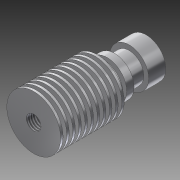
# Autodesk Inventor part: SINK-B
Saved by Autodesk Inventor 2014 SP1 (Build 180222100, 222)
## iProperties
Created: 2017-07-08
Part Number: SINK-B
Material: Типовые
Document SubType Name: Modeling
Designer: Stepan
Density: 1 g/cm^3
Appearance: Алюминий — полированный
Author: Stepan
Autodesk Inventor part; units mm, degrees
ref_plane "YZ Plane" through (0, 0, 0) normal (1, 0, 0) x (0, 1, 0)
ref_plane "XZ Plane" through (0, 0, 0) normal (0, 1, 0) x (-1, 0, 0)
ref_plane "XY Plane" through (0, 0, 0) normal (0, 0, 1) x (1, 0, 0)
sketch "Эскиз1" plane through (0, 0, 0) normal (0, 0, 1) x (1, 0, 0)
  line L0 (0, 46) -> (8, 46) construction
  line L1 (8, 46) -> (8, 39)
  line L2 (8, 39) -> (6, 39)
  line L3 (6, 39) -> (6, 33)
  line L4 (6, 33) -> (8, 33)
  line L5 (8, 33) -> (8, 30)
  line L6 (0, 0) -> (11.0018, 0)
  line L7 (11.0018, 0) -> (11.0018, 1)
  line L8 (11.0018, 1) -> (4, 1)
  line L9 (4, 1) -> (4, 2.5)
  line L10 (0, 2.5) -> (11, 2.5) construction
  line L11 (4, 2.5) -> (11, 2.5)
  line L12 (11, 2.5) -> (11, 3.5)
  line L13 (11, 3.5) -> (4, 3.5)
  line L14 (4, 3.5) -> (4, 5)
  line L15 (4, 21) -> (4, 22.5)
  line L16 (4, 22.5) -> (11, 22.5)
  line L17 (11, 22.5) -> (11, 23.5)
  line L18 (11, 23.5) -> (4, 23.5)
  line L19 (4, 23.5) -> (4, 25)
  line L20 (4, 25) -> (11, 25)
  line L21 (11, 25) -> (11, 26)
  line L22 (11, 26) -> (4, 26)
  line L23 (4, 26) -> (4, 27.5)
  line L24 (4, 27.5) -> (8, 27.5)
  line L25 (8, 27.5) -> (8, 28.5)
  line L26 (8, 28.5) -> (4, 28.5)
  line L27 (4, 28.5) -> (4, 30)
  line L28 (4, 30) -> (8, 30)
  line L29 (8, 46) -> (0, 46)
  line L30 (0, 0) -> (0, 46) construction
  line L31 (0, 0) -> (0, 46)
  line L32 (4, 21) -> (11, 21)
  line L33 (11, 21) -> (11, 20)
  line L34 (11, 20) -> (4, 20)
  line L35 (4, 20) -> (4, 18.5)
  line L36 (4, 18.5) -> (11, 18.5)
  line L37 (11, 18.5) -> (11, 17.5)
  line L38 (11, 17.5) -> (4, 17.5)
  line L39 (4, 17.5) -> (4, 16)
  line L40 (4, 16) -> (11, 16)
  line L41 (11, 16) -> (11, 15)
  line L42 (11, 15) -> (4, 15)
  line L43 (4, 15) -> (4, 13.5)
  line L44 (4, 13.5) -> (11, 13.5)
  line L45 (11, 13.5) -> (11, 12.5)
  line L46 (11, 12.5) -> (4, 12.5)
  line L47 (4, 12.5) -> (4, 11)
  line L48 (4, 11) -> (11, 11)
  line L49 (11, 11) -> (11, 10)
  line L50 (11, 10) -> (4, 10)
  line L51 (4, 10) -> (4, 8.5)
  line L52 (4, 8.5) -> (11, 8.5)
  line L53 (11, 8.5) -> (11, 7.5)
  line L54 (11, 7.5) -> (4, 7.5)
  line L55 (4, 7.5) -> (4, 6)
  line L56 (4, 6) -> (11, 6)
  line L57 (11, 6) -> (11, 5)
  line L58 (11, 5) -> (4, 5)
  dimension "d0" = 46
  dimension "d1" = 8
  dimension "d2" = 7
  dimension "d4" = 6
  dimension "d5" = 3
  dimension "d9" = 1
  dimension "d10" = 1.5
  dimension "d11" = 11
  dimension "d12" = 1
  dimension "d13" = 1.5
  dimension "d27" = 1.5
  dimension "d28" = 1
  dimension "d29" = 1.5
  dimension "d30" = 1.5
  dimension "d31" = 1
  dimension "d32" = 1
  dimension "d33" = 1.5
  dimension "d34" = 1
  dimension "d35" = 1.5
  dimension "d36" = 1
  dimension "d37" = 1.5
  dimension "d38" = 1
  dimension "d39" = 1.5
  dimension "d40" = 1
  dimension "d41" = 1.5
  dimension "d42" = 1
  dimension "d43" = 1.5
  constraints: 118 end point, 24 parallel, 20 perpendicular, 7 collinear
  measures "d0" distance of L6.start L0.start
  measures "d1" distance of L0.start L0.end
  measures "d2" distance of L0.end L1.end
  measures "d4" distance of L2.end L3.end
  measures "d5" distance of L4.end L5.end
  measures "d9" distance of L6.end L7.end
  measures "d10" distance of L8.end L9.end
  measures "d11" distance of L10.start L10.end
  measures "d12" distance of L10.end L12.end
  measures "d13" distance of L13.end L14.end
  measures "d27" distance of L15.start L15.end
  measures "d28" distance of L16.end L17.end
  measures "d29" distance of L18.end L19.end
  measures "d30" distance of L22.end L23.end
  measures "d31" distance of L24.end L25.end
  measures "d32" distance of L32.end L33.end
  measures "d33" distance of L34.end L35.end
  measures "d34" distance of L36.end L37.end
  measures "d35" distance of L38.end L39.end
  measures "d36" distance of L40.end L41.end
  measures "d37" distance of L42.end L43.end
  measures "d38" distance of L44.end L45.end
  measures "d39" distance of L46.end L47.end
  measures "d40" distance of L48.end L49.end
  measures "d41" distance of L50.end L51.end
  measures "d42" distance of L52.end L53.end
  measures "d43" distance of L54.end L55.end
revolve "Вращение1" add sketch "Эскиз1" angle 360 about axis through (0, 0, 0) along (0, 1, 0)
sketch "Эскиз2" plane through (0, 0, 0) normal (0, -1, 0) x (1, 0, 0)
  circle A0 centre (0, 0) radius 11.0018 projected
  circle A1 centre (0, 0) radius 3
  dimension "d45" = 6
  constraints: 1 centre point, 1 coincident
  measures "d45" diameter of A1
extrude "Выдавливание1" cut sketch "Эскиз2" against normal blind 13 contours A1
sketch "Эскиз3" plane through (0, 13, 0) normal (0, -1, 0) x (1, 0, 0)
  circle A0 centre (0, 0) radius 3 projected
  circle A1 centre (0, 0) radius 2.5
  dimension "d48" = 5
  constraints: 1 centre point, 1 coincident
  measures "d48" diameter of A1
extrude "Выдавливание2" cut sketch "Эскиз3" against normal blind 5 contours A1
sketch "Эскиз4" plane through (0, 18, 0) normal (0, -1, 0) x (1, 0, 0)
  circle A0 centre (0, 0) radius 2.5 projected
  circle A1 centre (0, 0) radius 1.6
  dimension "d51" = 3.2
  constraints: 1 centre point, 1 coincident
  measures "d51" diameter of A1
extrude "Выдавливание3" cut sketch "Эскиз4" against normal blind 12.75 contours A1
thread "Резьба1" size "M6x1" class "6H" standard "ANSI Metric M Profile" full length
sketch "Эскиз5" plane through (0, 46, 0) normal (0, 1, 0) x (1, 0, 0)
  circle A0 centre (0, 0) radius 8 projected
  circle A1 centre (0, 0) radius 6.5
  dimension "d56" = 13
  constraints: 1 centre point, 1 coincident
  measures "d56" diameter of A1
extrude "Выдавливание4" cut sketch "Эскиз5" against normal blind 5 contours A1
sketch "Эскиз6" plane through (0, 41, 0) normal (0, 1, 0) x (1, 0, 0)
  circle A0 centre (0, 0) radius 6.5 projected
  circle A1 centre (0, 0) radius 5
  dimension "d59" = 10
  constraints: 1 centre point, 1 coincident
  measures "d59" diameter of A1
extrude "Выдавливание5" cut sketch "Эскиз6" against normal blind 4 contours A1
chamfer "Фаска1" distance 1.5 angle 30 1 edges at (-5, 41, 0) measured on face at (-5.5, 41, 0)
sketch "Эскиз7" plane through (0, 37, 0) normal (0, 1, 0) x (1, 0, 0)
  circle A0 centre (0, 0) radius 5 projected
  circle A1 centre (0, 0) radius 3
  dimension "d65" = 6
  constraints: 1 centre point, 1 coincident
  measures "d65" diameter of A1
extrude "Выдавливание6" cut sketch "Эскиз7" against normal up to surface (6.25 mm away) contours A1
chamfer "Фаска2" distance 2 angle 30 1 edges at (-5, 37, 0) measured on face at (-4.5, 37, 0)
chamfer "Фаска3" distance 1.4 angle 30 1 edges at (-3, 30.75, 0) measured on face at (-2.5, 30.75, 0)
chamfer "Фаска4" distance 0.9 angle 35 1 edges at (-1.6, 18, 0) measured on face at (-2.1, 18, 0)
